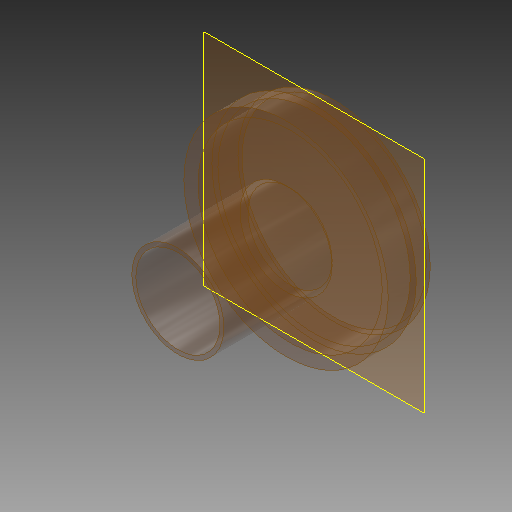
# Autodesk Inventor part: Bocal de Saída
Saved by Autodesk Inventor 2019 (Build 230136000, 136)
## iProperties
Created: 2020-04-02
Part Number: Bocal de Saída
Material: Genérico
Document SubType Name: Modeling
Designer: Paulo Rodrigues
Density: 1 g/cm^3
Appearance: Policarbonato - Fumê
Author: Paulo Rodrigues
Autodesk Inventor part; units mm, degrees
ref_plane "YZ Plane" through (0, 0, 0) normal (1, 0, 0) x (0, 1, 0)
ref_plane "XZ Plane" through (0, 0, 0) normal (0, 1, 0) x (-1, 0, 0)
ref_plane "XY Plane" through (0, 0, 0) normal (0, 0, 1) x (1, 0, 0)
ref_plane "Plano de trabalho1" through (0, 0, 0) normal (0, 0, 1) x (1, 0, 0)
sketch "Esboço1" plane through (0, 0, 0) normal (0, 0, 1) x (1, 0, 0)
  circle A0 centre (0, 0) radius 24 projected
  circle A1 centre (0, 0) radius 23
  point P0 (0, 0)
  dimension "d0" = 1
  constraints: 1 centre point
  measures "d0" radial gap between concentric circles of A0 A1
extrude "Extrusão1" add sketch "Esboço1" against normal blind 5
sketch "Esboço2" plane through (0, 0, 0) normal (0, 0, 1) x (1, 0, 0)
  circle A0 centre (0, 0) radius 23 projected
  circle A1 centre (0, 0) radius 25.5
  point P0 (0, 0)
  dimension "d3" = 2.5
  constraints: 1 centre point
  measures "d3" radial gap between concentric circles of A1 A0
extrude "Extrusão2" add sketch "Esboço2" along normal blind 7
sketch "Esboço3" plane through (0, 0, 7) normal (0, 0, 1) x (1, 0, 0)
  circle A0 centre (0, 0) radius 23 projected
  point P0 (0, 0)
extrude "Extrusão3" add sketch "Esboço3" against normal blind 1
sketch "Esboço4" plane through (0, 0, 7) normal (0, 0, 1) x (1, 0, 0)
  circle A0 centre (0, 0) radius 11.5
  dimension "d8" = 23
  constraints: 1 centre point, 1 coincident
  measures "d8" diameter of A0
extrude "Extrusão4" add sketch "Esboço4" along normal blind 27
sketch "Esboço5" plane through (0, 0, 34) normal (0, 0, 1) x (1, 0, 0)
  circle A0 centre (0, 0) radius 11.5 projected
  circle A1 centre (0, 0) radius 10.5
  dimension "d11" = 1
  constraints: 1 centre point
  measures "d11" radial gap between concentric circles of A0 A1
extrude "Extrusão5" cut sketch "Esboço5" against normal through all contours A1
